Autodesk Inventor part; units mm, degrees
(part 2 of 4)
  line L999 (8.8018, 62.5401) -> (8.8176, 62.5237)
  line L1000 (8.788, 62.5566) -> (8.8018, 62.5401)
  line L1001 (8.7764, 62.5733) -> (8.788, 62.5566)
  line L1002 (8.7669, 62.5901) -> (8.7764, 62.5733)
  line L1003 (8.7595, 62.6071) -> (8.7669, 62.5901)
  line L1004 (8.7542, 62.6241) -> (8.7595, 62.6071)
  line L1005 (8.7511, 62.6412) -> (8.7542, 62.6241)
  line L1006 (8.75, 62.6584) -> (8.7511, 62.6412)
  line L1007 (8.75, 62.8319) -> (8.75, 62.6584)
  line L1008 (8.8777, 62.4763) -> (8.9019, 62.461)
  line L1009 (8.9019, 62.461) -> (8.9282, 62.4462)
  line L1010 (8.9282, 62.4462) -> (8.9566, 62.4317)
  line L1011 (8.9566, 62.4317) -> (8.9871, 62.4176)
  line L1012 (9.0196, 62.4039) -> (9.0542, 62.3907)
  line L1013 (8.9871, 62.4176) -> (9.0196, 62.4039)
  line L1014 (8.7764, 59.9488) -> (8.788, 59.9655)
  line L1015 (8.788, 59.9655) -> (8.8018, 59.9821)
  line L1016 (8.8018, 59.9821) -> (8.8176, 59.9984)
  line L1017 (8.8176, 59.9984) -> (8.8355, 60.0145)
  line L1018 (8.8355, 60.0145) -> (8.8556, 60.0303)
  line L1019 (8.8556, 60.0303) -> (8.8777, 60.0458)
  line L1020 (8.8777, 60.0458) -> (8.9019, 60.0611)
  line L1021 (8.9019, 60.0611) -> (8.9282, 60.0759)
  line L1022 (8.9282, 60.0759) -> (8.9566, 60.0904)
  line L1023 (8.9566, 60.0904) -> (8.9871, 60.1045)
  line L1024 (8.9871, 60.1045) -> (9.0196, 60.1182)
  line L1025 (9.0196, 60.1182) -> (9.0542, 60.1314)
  line L1026 (8.7669, 59.932) -> (8.7764, 59.9488)
  line L1027 (8.7595, 59.915) -> (8.7669, 59.932)
  line L1028 (8.7542, 59.898) -> (8.7595, 59.915)
  line L1029 (8.7511, 59.8809) -> (8.7542, 59.898)
  line L1030 (8.75, 59.8637) -> (8.7511, 59.8809)
  line L1031 (8.75, 59.6903) -> (8.75, 59.8637)
  line L1032 (8.75, 59.6903) -> (8.75, 59.5168)
  line L1033 (8.75, 59.5168) -> (8.7511, 59.4996)
  line L1034 (8.7511, 59.4996) -> (8.7542, 59.4825)
  line L1035 (8.7542, 59.4825) -> (8.7595, 59.4655)
  line L1036 (8.7595, 59.4655) -> (8.7669, 59.4485)
  line L1037 (8.7669, 59.4485) -> (8.7764, 59.4317)
  line L1038 (8.7764, 59.4317) -> (8.788, 59.415)
  line L1039 (8.788, 59.415) -> (8.8018, 59.3985)
  line L1040 (8.8018, 59.3985) -> (8.8176, 59.3821)
  line L1041 (8.8176, 59.3821) -> (8.8355, 59.366)
  line L1042 (8.8556, 59.3502) -> (8.8777, 59.3347)
  line L1043 (8.8355, 59.366) -> (8.8556, 59.3502)
  line L1044 (8.8777, 59.3347) -> (8.9019, 59.3195)
  line L1045 (8.9019, 59.3195) -> (8.9282, 59.3046)
  line L1046 (8.9282, 59.3046) -> (8.9566, 59.2901)
  line L1047 (8.9566, 59.2901) -> (8.9871, 59.276)
  line L1048 (8.9871, 59.276) -> (9.0196, 59.2623)
  line L1049 (9.0196, 59.2623) -> (9.0542, 59.2491)
  line L1050 (9.0542, 59.2491) -> (11, 58.5409)
  line L1051 (11, 58.5409) -> (11, 58.1195)
  line L1052 (9.0542, 56.9898) -> (11, 57.698)
  line L1053 (11, 57.698) -> (11, 58.1195)
  line L1054 (8.8018, 56.8405) -> (8.8176, 56.8568)
  line L1055 (8.8176, 56.8568) -> (8.8355, 56.8729)
  line L1056 (8.8355, 56.8729) -> (8.8556, 56.8887)
  line L1057 (8.8556, 56.8887) -> (8.8777, 56.9043)
  line L1058 (8.8777, 56.9043) -> (8.9019, 56.9195)
  line L1059 (8.9019, 56.9195) -> (8.9282, 56.9344)
  line L1060 (8.9282, 56.9344) -> (8.9566, 56.9489)
  line L1061 (8.9566, 56.9489) -> (8.9871, 56.963)
  line L1062 (8.9871, 56.963) -> (9.0196, 56.9766)
  line L1063 (9.0196, 56.9766) -> (9.0542, 56.9898)
  line L1064 (8.75, 56.5487) -> (8.75, 56.7222)
  line L1065 (8.75, 56.7222) -> (8.7511, 56.7393)
  line L1066 (8.7511, 56.7393) -> (8.7542, 56.7564)
  line L1067 (8.7542, 56.7564) -> (8.7595, 56.7734)
  line L1068 (8.7595, 56.7734) -> (8.7669, 56.7904)
  line L1069 (8.7669, 56.7904) -> (8.7764, 56.8072)
  line L1070 (8.7764, 56.8072) -> (8.788, 56.8239)
  line L1071 (8.788, 56.8239) -> (8.8018, 56.8405)
  line L1072 (8.8777, 56.1931) -> (8.9019, 56.1779)
  line L1073 (8.9019, 56.1779) -> (8.9282, 56.163)
  line L1074 (8.9282, 56.163) -> (8.9566, 56.1485)
  line L1075 (8.9566, 56.1485) -> (8.9871, 56.1344)
  line L1076 (8.7595, 56.3239) -> (8.7669, 56.3069)
  line L1077 (8.7669, 56.3069) -> (8.7764, 56.2901)
  line L1078 (8.7764, 56.2901) -> (8.788, 56.2734)
  line L1079 (8.75, 56.5487) -> (8.75, 56.3752)
  line L1080 (8.75, 56.3752) -> (8.7511, 56.358)
  line L1081 (8.7511, 56.358) -> (8.7542, 56.3409)
  line L1082 (8.7542, 56.3409) -> (8.7595, 56.3239)
  line L1083 (8.788, 56.2734) -> (8.8018, 56.2569)
  line L1084 (8.8018, 56.2569) -> (8.8176, 56.2405)
  line L1085 (8.8355, 56.2245) -> (8.8556, 56.2086)
  line L1086 (8.8556, 56.2086) -> (8.8777, 56.1931)
  line L1087 (8.8176, 56.2405) -> (8.8355, 56.2245)
  line L1088 (8.9871, 56.1344) -> (9.0196, 56.1207)
  line L1089 (9.0196, 56.1207) -> (9.0542, 56.1075)
  line L1090 (9.0542, 56.1075) -> (11, 55.3993)
  line L1091 (11, 55.3993) -> (11, 54.9779)
  line L1092 (9.0542, 53.8482) -> (11, 54.5564)
  line L1093 (11, 54.5564) -> (11, 54.9779)
  line L1094 (8.8777, 53.7627) -> (8.9019, 53.7779)
  line L1095 (8.9019, 53.7779) -> (8.9282, 53.7928)
  line L1096 (8.9282, 53.7928) -> (8.9566, 53.8073)
  line L1097 (8.9566, 53.8073) -> (8.9871, 53.8214)
  line L1098 (8.9871, 53.8214) -> (9.0196, 53.835)
  line L1099 (9.0196, 53.835) -> (9.0542, 53.8482)
  line L1100 (9.0196, 52.9791) -> (9.0542, 52.9659)
  line L1101 (8.9871, 52.9928) -> (9.0196, 52.9791)
  line L1102 (8.9566, 53.0069) -> (8.9871, 52.9928)
  line L1103 (8.9019, 53.0363) -> (8.9282, 53.0214)
  line L1104 (8.8777, 53.0515) -> (8.9019, 53.0363)
  line L1105 (8.8355, 53.0829) -> (8.8556, 53.067)
  line L1106 (8.8176, 53.099) -> (8.8355, 53.0829)
  line L1107 (8.9282, 53.0214) -> (8.9566, 53.0069)
  line L1108 (8.75, 50.2655) -> (8.75, 50.439)
  line L1109 (8.75, 50.439) -> (8.7511, 50.4561)
  line L1110 (8.7511, 50.4561) -> (8.7542, 50.4732)
  line L1111 (8.7542, 50.4732) -> (8.7595, 50.4903)
  line L1112 (8.7595, 50.4903) -> (8.7669, 50.5072)
  line L1113 (8.7669, 50.5072) -> (8.7764, 50.5241)
  line L1114 (8.7764, 50.5241) -> (8.788, 50.5408)
  line L1115 (8.8556, 50.6055) -> (8.8777, 50.6211)
  line L1116 (8.8355, 50.5897) -> (8.8556, 50.6055)
  line L1117 (8.8176, 50.5736) -> (8.8355, 50.5897)
  line L1118 (8.8018, 50.5573) -> (8.8176, 50.5736)
  line L1119 (8.788, 50.5408) -> (8.8018, 50.5573)
  line L1120 (8.8556, 53.067) -> (8.8777, 53.0515)
  line L1121 (9.0542, 60.1314) -> (11, 60.8396)
  line L1122 (11, 60.8396) -> (11, 61.2611)
  line L1123 (11, 61.6825) -> (11, 61.2611)
  line L1124 (9.0542, 62.3907) -> (11, 61.6825)
  line L1125 (8.9282, 88.3503) -> (8.9566, 88.3648)
  line L1126 (8.9566, 88.3648) -> (8.9871, 88.3789)
  line L1127 (8.9871, 88.3789) -> (9.0196, 88.3925)
  line L1128 (8.7669, 88.2063) -> (8.7764, 88.2232)
  line L1129 (8.7764, 88.2232) -> (8.788, 88.2399)
  line L1130 (8.788, 88.2399) -> (8.8018, 88.2564)
  line L1131 (8.8018, 88.2564) -> (8.8176, 88.2727)
  line L1132 (8.8176, 88.2727) -> (8.8355, 88.2888)
  line L1133 (8.8355, 88.2888) -> (8.8556, 88.3046)
  line L1134 (8.8556, 88.3046) -> (8.8777, 88.3202)
  line L1135 (8.8777, 88.3202) -> (8.9019, 88.3354)
  line L1136 (8.9019, 88.3354) -> (8.9282, 88.3503)
  line L1137 (8.75, 87.9646) -> (8.75, 88.1381)
  line L1138 (8.75, 88.1381) -> (8.7511, 88.1552)
  line L1139 (8.7542, 88.1723) -> (8.7595, 88.1894)
  line L1140 (8.7511, 88.1552) -> (8.7542, 88.1723)
  line L1141 (8.75, 87.9646) -> (8.75, 87.7911)
  line L1142 (8.75, 87.7911) -> (8.7511, 87.774)
  line L1143 (8.7511, 87.774) -> (8.7542, 87.7569)
  line L1144 (8.7542, 87.7569) -> (8.7595, 87.7398)
  line L1145 (8.7595, 87.7398) -> (8.7669, 87.7229)
  line L1146 (8.7669, 87.7229) -> (8.7764, 87.706)
  line L1147 (8.7595, 88.1894) -> (8.7669, 88.2063)
  line L1148 (8.9566, 87.5644) -> (8.9871, 87.5503)
  line L1149 (8.9871, 87.5503) -> (9.0196, 87.5366)
  line L1150 (9.0196, 87.5366) -> (9.0542, 87.5234)
  line L1151 (9.0542, 85.2642) -> (11, 85.9724)
  line L1152 (9.0542, 87.5234) -> (11, 86.8152)
  line L1153 (11, 85.9724) -> (11, 86.3938)
  line L1154 (11, 86.8152) -> (11, 86.3938)
  line L1155 (8.9282, 87.5789) -> (8.9566, 87.5644)
  line L1156 (8.9019, 87.5938) -> (8.9282, 87.5789)
  line L1157 (8.8777, 87.609) -> (8.9019, 87.5938)
  line L1158 (8.8556, 87.6246) -> (8.8777, 87.609)
  line L1159 (8.8355, 87.6404) -> (8.8556, 87.6246)
  line L1160 (8.8176, 87.6565) -> (8.8355, 87.6404)
  line L1161 (8.8018, 87.6728) -> (8.8176, 87.6565)
  line L1162 (8.7764, 87.706) -> (8.788, 87.6893)
  line L1163 (8.788, 87.6893) -> (8.8018, 87.6728)
  line L1164 (8.8018, 85.1148) -> (8.8176, 85.1311)
  line L1165 (8.788, 85.0983) -> (8.8018, 85.1148)
  line L1166 (8.7764, 85.0816) -> (8.788, 85.0983)
  line L1167 (8.7669, 85.0647) -> (8.7764, 85.0816)
  line L1168 (8.7595, 85.0478) -> (8.7669, 85.0647)
  line L1169 (8.7511, 85.0136) -> (8.7542, 85.0307)
  line L1170 (8.75, 84.9965) -> (8.7511, 85.0136)
  line L1171 (8.75, 84.823) -> (8.75, 84.9965)
  line L1172 (8.7542, 85.0307) -> (8.7595, 85.0478)
  line L1173 (8.75, 84.823) -> (8.75, 84.6495)
  line L1174 (8.75, 84.6495) -> (8.7511, 84.6324)
  line L1175 (8.7511, 84.6324) -> (8.7542, 84.6153)
  line L1176 (8.7542, 84.6153) -> (8.7595, 84.5982)
  line L1177 (8.7595, 84.5982) -> (8.7669, 84.5813)
  line L1178 (8.7669, 84.5813) -> (8.7764, 84.5644)
  line L1179 (8.7764, 84.5644) -> (8.788, 84.5477)
  line L1180 (8.788, 84.5477) -> (8.8018, 84.5312)
  line L1181 (8.8018, 84.5312) -> (8.8176, 84.5149)
  line L1182 (8.8355, 84.4988) -> (8.8556, 84.483)
  line L1183 (8.8556, 84.483) -> (8.8777, 84.4674)
  line L1184 (8.8777, 84.4674) -> (8.9019, 84.4522)
  line L1185 (8.9019, 84.4522) -> (8.9282, 84.4373)
  line L1186 (8.9282, 84.4373) -> (8.9566, 84.4228)
  line L1187 (8.8176, 84.5149) -> (8.8355, 84.4988)
  line L1188 (8.9871, 84.4087) -> (9.0196, 84.395)
  line L1189 (9.0196, 84.395) -> (9.0542, 84.3818)
  line L1190 (9.0542, 84.3818) -> (11, 83.6736)
  line L1191 (11, 83.6736) -> (11, 83.2522)
  line L1192 (11, 82.8308) -> (11, 83.2522)
  line L1193 (9.0542, 82.1226) -> (11, 82.8308)
  line L1194 (8.9566, 84.4228) -> (8.9871, 84.4087)
  line L1195 (8.8777, 82.037) -> (8.9019, 82.0522)
  line L1196 (8.9019, 82.0522) -> (8.9282, 82.0671)
  line L1197 (8.9282, 82.0671) -> (8.9566, 82.0816)
  line L1198 (8.9871, 82.0957) -> (9.0196, 82.1094)
  line L1199 (9.0196, 82.1094) -> (9.0542, 82.1226)
  line L1200 (8.9566, 82.0816) -> (8.9871, 82.0957)
  line L1201 (8.75, 81.6814) -> (8.75, 81.8549)
  line L1202 (8.75, 81.8549) -> (8.7511, 81.872)
  line L1203 (8.7511, 81.872) -> (8.7542, 81.8891)
  line L1204 (8.7542, 81.8891) -> (8.7595, 81.9062)
  line L1205 (8.7595, 81.9062) -> (8.7669, 81.9231)
  line L1206 (8.7669, 81.9231) -> (8.7764, 81.94)
  line L1207 (8.7764, 81.94) -> (8.788, 81.9567)
  line L1208 (8.788, 81.9567) -> (8.8018, 81.9732)
  line L1209 (8.8018, 81.9732) -> (8.8176, 81.9895)
  line L1210 (8.8176, 81.9895) -> (8.8355, 82.0056)
  line L1211 (8.8355, 82.0056) -> (8.8556, 82.0215)
  line L1212 (8.8556, 82.0215) -> (8.8777, 82.037)
  line L1213 (8.8777, 81.3258) -> (8.9019, 81.3106)
  line L1214 (8.9019, 81.3106) -> (8.9282, 81.2957)
  line L1215 (8.75, 81.6814) -> (8.75, 81.5079)
  line L1216 (8.75, 81.5079) -> (8.7511, 81.4908)
  line L1217 (8.7511, 81.4908) -> (8.7542, 81.4737)
  line L1218 (8.7542, 81.4737) -> (8.7595, 81.4566)
  line L1219 (8.8556, 81.3414) -> (8.8777, 81.3258)
  line L1220 (8.8355, 81.3572) -> (8.8556, 81.3414)
  line L1221 (8.8176, 81.3733) -> (8.8355, 81.3572)
  line L1222 (8.7669, 81.4397) -> (8.7764, 81.4228)
  line L1223 (8.7764, 81.4228) -> (8.788, 81.4061)
  line L1224 (8.788, 81.4061) -> (8.8018, 81.3896)
  line L1225 (8.8018, 81.3896) -> (8.8176, 81.3733)
  line L1226 (8.7595, 81.4566) -> (8.7669, 81.4397)
  line L1227 (9.0196, 81.2535) -> (9.0542, 81.2402)
  line L1228 (8.9871, 81.2671) -> (9.0196, 81.2535)
  line L1229 (8.9282, 81.2957) -> (8.9566, 81.2812)
  line L1230 (8.9566, 81.2812) -> (8.9871, 81.2671)
  line L1231 (8.9871, 78.9541) -> (9.0196, 78.9678)
  line L1232 (9.0196, 78.9678) -> (9.0542, 78.981)
  line L1233 (9.0542, 78.981) -> (11, 79.6892)
  line L1234 (11, 79.6892) -> (11, 80.1106)
  line L1235 (11, 80.532) -> (11, 80.1106)
  line L1236 (9.0542, 81.2402) -> (11, 80.532)
  line L1237 (8.9566, 78.94) -> (8.9871, 78.9541)
  line L1238 (8.7764, 78.7984) -> (8.788, 78.8151)
  line L1239 (8.8018, 78.8316) -> (8.8176, 78.8479)
  line L1240 (8.8176, 78.8479) -> (8.8355, 78.864)
  line L1241 (8.8355, 78.864) -> (8.8556, 78.8799)
  line L1242 (8.8556, 78.8799) -> (8.8777, 78.8954)
  line L1243 (8.8777, 78.8954) -> (8.9019, 78.9106)
  line L1244 (8.9019, 78.9106) -> (8.9282, 78.9255)
  line L1245 (8.9282, 78.9255) -> (8.9566, 78.94)
  line L1246 (8.788, 78.8151) -> (8.8018, 78.8316)
  line L1247 (8.75, 78.5398) -> (8.75, 78.7133)
  line L1248 (8.75, 78.7133) -> (8.7511, 78.7304)
  line L1249 (8.7511, 78.7304) -> (8.7542, 78.7475)
  line L1250 (8.7595, 78.7646) -> (8.7669, 78.7815)
  line L1251 (8.7669, 78.7815) -> (8.7764, 78.7984)
  line L1252 (8.7542, 78.7475) -> (8.7595, 78.7646)
  line L1253 (8.788, 78.2645) -> (8.8018, 78.248)
  line L1254 (8.7764, 78.2812) -> (8.788, 78.2645)
  line L1255 (8.7669, 78.2981) -> (8.7764, 78.2812)
  line L1256 (8.7595, 78.315) -> (8.7669, 78.2981)
  line L1257 (8.7542, 78.3321) -> (8.7595, 78.315)
  line L1258 (8.7511, 78.3492) -> (8.7542, 78.3321)
  line L1259 (8.75, 78.3663) -> (8.7511, 78.3492)
  line L1260 (8.75, 78.5398) -> (8.75, 78.3663)
  line L1261 (8.9871, 75.8125) -> (9.0196, 75.8262)
  line L1262 (9.0196, 75.8262) -> (9.0542, 75.8394)
  line L1263 (9.0542, 75.8394) -> (11, 76.5476)
  line L1264 (11, 76.5476) -> (11, 76.969)
  line L1265 (11, 77.3904) -> (11, 76.969)
  line L1266 (9.0542, 78.0987) -> (11, 77.3904)
  line L1267 (9.0196, 78.1119) -> (9.0542, 78.0987)
  line L1268 (8.8018, 78.248) -> (8.8176, 78.2317)
  line L1269 (8.8176, 78.2317) -> (8.8355, 78.2156)
  line L1270 (8.8355, 78.2156) -> (8.8556, 78.1998)
  line L1271 (8.8556, 78.1998) -> (8.8777, 78.1842)
  line L1272 (8.8777, 78.1842) -> (8.9019, 78.169)
  line L1273 (8.9019, 78.169) -> (8.9282, 78.1541)
  line L1274 (8.9282, 78.1541) -> (8.9566, 78.1396)
  line L1275 (8.9566, 78.1396) -> (8.9871, 78.1255)
  line L1276 (8.9871, 78.1255) -> (9.0196, 78.1119)
  line L1277 (8.8176, 85.1311) -> (8.8355, 85.1472)
  line L1278 (8.8355, 85.1472) -> (8.8556, 85.163)
  line L1279 (8.8556, 85.163) -> (8.8777, 85.1786)
  line L1280 (8.8777, 85.1786) -> (8.9019, 85.1938)
  line L1281 (8.9019, 85.1938) -> (8.9282, 85.2087)
  line L1282 (8.9282, 85.2087) -> (8.9566, 85.2232)
  line L1283 (8.9566, 85.2232) -> (8.9871, 85.2373)
  line L1284 (8.9871, 85.2373) -> (9.0196, 85.251)
  line L1285 (9.0196, 85.251) -> (9.0542, 85.2642)
  line L1286 (-1.25, 99.281) -> (-1.25, 109.281)
  line L1287 (-1.25, 109.281) -> (8.75, 109.281)
  line L1288 (8.75, 109.281) -> (8.75, 100.531)
  line L1289 (9.6684, 106.1616) -> (10.0504, 106.1616)
  line L1290 (10.0504, 106.1616) -> (10.0504, 106.0668)
  line L1291 (10.0504, 106.0668) -> (9.6684, 106.0668)
  line L1292 (9.6684, 106.0668) -> (9.6684, 106.1616)
  line L1293 (-2.25, 0) -> (-1.25, 0)
  line L1294 (8.75, 0) -> (12, 0)
  line L1295 (-1.25, 99.281) -> (-1.25, 10.75)
  line L1296 (8.7511, -56.358) -> (8.7542, -56.3409)
  line L1297 (8.7542, -56.3409) -> (8.7595, -56.3239)
  line L1298 (8.7595, -56.3239) -> (8.7669, -56.3069)
  line L1299 (8.7669, -56.3069) -> (8.7764, -56.2901)
  line L1300 (8.7764, -56.2901) -> (8.788, -56.2734)
  line L1301 (8.788, -56.2734) -> (8.8018, -56.2569)
  line L1302 (8.8018, -56.2569) -> (8.8176, -56.2405)
  line L1303 (8.8176, -56.2405) -> (8.8355, -56.2245)
  line L1304 (8.8355, -56.2245) -> (8.8556, -56.2086)
  line L1305 (8.8556, -56.2086) -> (8.8777, -56.1931)
  line L1306 (8.8777, -56.1931) -> (8.9019, -56.1779)
  line L1307 (8.9019, -56.1779) -> (8.9282, -56.163)
  line L1308 (8.9282, -56.163) -> (8.9566, -56.1485)
  line L1309 (8.9566, -56.1485) -> (8.9871, -56.1344)
  line L1310 (8.788, -56.8239) -> (8.8018, -56.8405)
  line L1311 (8.7764, -56.8072) -> (8.788, -56.8239)
  line L1312 (8.7669, -56.7904) -> (8.7764, -56.8072)
  line L1313 (8.7595, -56.7734) -> (8.7669, -56.7904)
  line L1314 (8.7542, -56.7564) -> (8.7595, -56.7734)
  line L1315 (8.75, -56.7222) -> (8.7511, -56.7393)
  line L1316 (8.75, -56.5487) -> (8.75, -56.7222)
  line L1317 (8.75, -56.5487) -> (8.75, -56.3752)
  line L1318 (8.75, -56.3752) -> (8.7511, -56.358)
  line L1319 (8.7511, -56.7393) -> (8.7542, -56.7564)
  line L1320 (9.0196, -56.9766) -> (9.0542, -56.9898)
  line L1321 (8.9871, -56.963) -> (9.0196, -56.9766)
  line L1322 (8.9566, -56.9489) -> (8.9871, -56.963)
  line L1323 (8.9282, -56.9344) -> (8.9566, -56.9489)
  line L1324 (8.9019, -56.9195) -> (8.9282, -56.9344)
  line L1325 (8.8777, -56.9043) -> (8.9019, -56.9195)
  line L1326 (8.8355, -56.8729) -> (8.8556, -56.8887)
  line L1327 (8.8176, -56.8568) -> (8.8355, -56.8729)
  line L1328 (8.8018, -56.8405) -> (8.8176, -56.8568)
  line L1329 (8.8556, -56.8887) -> (8.8777, -56.9043)
  line L1330 (8.8018, -59.3985) -> (8.8176, -59.3821)
  line L1331 (8.8176, -59.3821) -> (8.8355, -59.366)
  line L1332 (8.8556, -59.3502) -> (8.8777, -59.3347)
  line L1333 (8.8355, -59.366) -> (8.8556, -59.3502)
  line L1334 (8.8777, -59.3347) -> (8.9019, -59.3195)
  line L1335 (8.9019, -59.3195) -> (8.9282, -59.3046)
  line L1336 (8.9282, -59.3046) -> (8.9566, -59.2901)
  line L1337 (9.0542, -56.9898) -> (11, -57.698)
  line L1338 (11, -57.698) -> (11, -58.1195)
  line L1339 (8.9566, -59.2901) -> (8.9871, -59.276)
  line L1340 (8.9871, -59.276) -> (9.0196, -59.2623)
  line L1341 (11, -58.5409) -> (11, -58.1195)
  line L1342 (9.0542, -59.2491) -> (11, -58.5409)
  line L1343 (9.0196, -59.2623) -> (9.0542, -59.2491)
  line L1344 (8.788, -59.415) -> (8.8018, -59.3985)
  line L1345 (8.7764, -59.4317) -> (8.788, -59.415)
  line L1346 (8.7669, -59.4485) -> (8.7764, -59.4317)
  line L1347 (8.7595, -59.4655) -> (8.7669, -59.4485)
  line L1348 (8.7542, -59.4825) -> (8.7595, -59.4655)
  line L1349 (8.7511, -59.4996) -> (8.7542, -59.4825)
  line L1350 (8.75, -59.5168) -> (8.7511, -59.4996)
  line L1351 (8.75, -59.6903) -> (8.75, -59.5168)
  line L1352 (8.75, -59.6903) -> (8.75, -59.8637)
  line L1353 (8.7511, -59.8809) -> (8.7542, -59.898)
  line L1354 (8.7542, -59.898) -> (8.7595, -59.915)
  line L1355 (8.7595, -59.915) -> (8.7669, -59.932)
  line L1356 (8.7669, -59.932) -> (8.7764, -59.9488)
  line L1357 (8.75, -59.8637) -> (8.7511, -59.8809)
  line L1358 (8.9871, -60.1045) -> (9.0196, -60.1182)
  line L1359 (8.9566, -60.0904) -> (8.9871, -60.1045)
  line L1360 (8.9282, -60.0759) -> (8.9566, -60.0904)
  line L1361 (8.9019, -60.0611) -> (8.9282, -60.0759)
  line L1362 (8.8777, -60.0458) -> (8.9019, -60.0611)
  line L1363 (8.8556, -60.0303) -> (8.8777, -60.0458)
  line L1364 (8.8355, -60.0145) -> (8.8556, -60.0303)
  line L1365 (8.8176, -59.9984) -> (8.8355, -60.0145)
  line L1366 (8.8018, -59.9821) -> (8.8176, -59.9984)
  line L1367 (8.788, -59.9655) -> (8.8018, -59.9821)
  line L1368 (8.7764, -59.9488) -> (8.788, -59.9655)
  line L1369 (8.7764, -63.0904) -> (8.788, -63.1071)
  line L1370 (8.8018, -63.1237) -> (8.8176, -63.14)
  line L1371 (8.8176, -63.14) -> (8.8355, -63.1561)
  line L1372 (8.788, -63.1071) -> (8.8018, -63.1237)
  line L1373 (8.8556, -62.4918) -> (8.8777, -62.4763)
  line L1374 (8.8355, -62.5076) -> (8.8556, -62.4918)
  line L1375 (8.8176, -62.5237) -> (8.8355, -62.5076)
  line L1376 (8.8018, -62.5401) -> (8.8176, -62.5237)
  line L1377 (8.788, -62.5566) -> (8.8018, -62.5401)
  line L1378 (8.7764, -62.5733) -> (8.788, -62.5566)
  line L1379 (8.7669, -62.5901) -> (8.7764, -62.5733)
  line L1380 (8.7542, -62.6241) -> (8.7595, -62.6071)
  line L1381 (8.7511, -62.6412) -> (8.7542, -62.6241)
  line L1382 (8.75, -62.6584) -> (8.7511, -62.6412)
  line L1383 (8.75, -62.8319) -> (8.75, -62.6584)
  line L1384 (8.7595, -62.6071) -> (8.7669, -62.5901)
  line L1385 (8.75, -65.9734) -> (8.75, -66.1469)
  line L1386 (8.75, -66.1469) -> (8.7511, -66.1641)
  line L1387 (8.7595, -68.8903) -> (8.7669, -68.8733)
  line L1388 (8.7542, -68.9073) -> (8.7595, -68.8903)
  line L1389 (8.7511, -68.9244) -> (8.7542, -68.9073)
  line L1390 (8.75, -68.9416) -> (8.7511, -68.9244)
  line L1391 (8.75, -69.115) -> (8.75, -68.9416)
  line L1392 (8.75, -75.3982) -> (7.9383, -75.3982)
  line L1393 (8.7669, -68.8733) -> (8.7764, -68.8565)
  line L1394 (8.7595, -90.8814) -> (8.7669, -90.8645)
  line L1395 (8.7511, -90.9156) -> (8.7542, -90.8985)
  line L1396 (8.7542, -90.8985) -> (8.7595, -90.8814)
  line L1397 (8.8777, -62.4763) -> (8.9019, -62.461)
  line L1398 (8.9019, -62.461) -> (8.9282, -62.4462)
  line L1399 (8.9282, -62.4462) -> (8.9566, -62.4317)
  line L1400 (8.9566, -62.4317) -> (8.9871, -62.4176)
  line L1401 (9.0196, -62.4039) -> (9.0542, -62.3907)
  line L1402 (9.0542, -60.1314) -> (11, -60.8396)
  line L1403 (8.9871, -62.4176) -> (9.0196, -62.4039)
  line L1404 (11, -60.8396) -> (11, -61.2611)
  line L1405 (11, -61.6825) -> (11, -61.2611)
  line L1406 (9.0542, -62.3907) -> (11, -61.6825)
  line L1407 (9.0196, -60.1182) -> (9.0542, -60.1314)
  line L1408 (8.8176, -12.2583) -> (8.8355, -12.2422)
  line L1409 (8.8018, -12.2746) -> (8.8176, -12.2583)
  line L1410 (8.788, -12.2911) -> (8.8018, -12.2746)
  line L1411 (8.7764, -12.3078) -> (8.788, -12.2911)
  line L1412 (8.7669, -12.3246) -> (8.7764, -12.3078)
  line L1413 (8.7595, -12.3416) -> (8.7669, -12.3246)
  line L1414 (8.7542, -12.3586) -> (8.7595, -12.3416)
  line L1415 (8.7511, -12.3758) -> (8.7542, -12.3586)
  line L1416 (8.75, -12.3929) -> (8.7511, -12.3758)
  line L1417 (8.75, -12.5664) -> (8.75, -12.3929)
  line L1418 (8.75, -12.5664) -> (7.1265, -12.5664)
  line L1419 (8.9282, -12.1807) -> (8.9566, -12.1662)
  line L1420 (8.9566, -12.1662) -> (8.9871, -12.1521)
  line L1421 (8.9871, -12.1521) -> (9.0196, -12.1384)
  line L1422 (9.0196, -12.1384) -> (9.0542, -12.1252)
  line L1423 (8.8355, -12.2422) -> (8.8556, -12.2263)
  line L1424 (8.8556, -12.2263) -> (8.8777, -12.2108)
  line L1425 (8.8777, -12.2108) -> (8.9019, -12.1956)
  line L1426 (8.9019, -12.1956) -> (8.9282, -12.1807)
  line L1427 (9.0542, -12.1252) -> (11, -11.417)
  line L1428 (11, -11.417) -> (11, -10.9956)
  line L1429 (8.75, -25.1327) -> (8.75, -24.9593)
  line L1430 (9.0542, -53.8482) -> (11, -54.5564)
  line L1431 (11, -54.5564) -> (11, -54.9779)
  line L1432 (9.0196, -56.1207) -> (9.0542, -56.1075)
  line L1433 (11, -55.3993) -> (11, -54.9779)
  line L1434 (9.0542, -56.1075) -> (11, -55.3993)
  line L1435 (8.9871, -56.1344) -> (9.0196, -56.1207)
  line L1436 (8.7542, -40.633) -> (8.7595, -40.6159)
  line L1437 (8.7511, -40.6501) -> (8.7542, -40.633)
  line L1438 (8.75, -40.6672) -> (8.7511, -40.6501)
  line L1439 (8.75, -40.8407) -> (8.75, -40.6672)
  line L1440 (8.75, -40.8407) -> (8.75, -41.0142)
  line L1441 (8.75, -41.0142) -> (8.7511, -41.0313)
  line L1442 (8.7511, -41.0313) -> (8.7542, -41.0484)
  line L1443 (8.7542, -41.0484) -> (8.7595, -41.0655)
  line L1444 (8.7542, -50.0578) -> (8.7595, -50.0407)
  line L1445 (8.75, -50.092) -> (8.7511, -50.0749)
  line L1446 (8.7764, -53.6656) -> (8.788, -53.6823)
  line L1447 (8.9871, -53.8214) -> (9.0196, -53.835)
  line L1448 (8.9566, -53.8073) -> (8.9871, -53.8214)
  line L1449 (8.9282, -53.7928) -> (8.9566, -53.8073)
  line L1450 (8.9019, -53.7779) -> (8.9282, -53.7928)
  line L1451 (8.8777, -53.7627) -> (8.9019, -53.7779)
  line L1452 (8.8556, -53.7471) -> (8.8777, -53.7627)
  line L1453 (8.8355, -53.7313) -> (8.8556, -53.7471)
  line L1454 (8.8176, -53.7152) -> (8.8355, -53.7313)
  line L1455 (8.8018, -53.6989) -> (8.8176, -53.7152)
  line L1456 (8.788, -53.6823) -> (8.8018, -53.6989)
  line L1457 (9.0196, -53.835) -> (9.0542, -53.8482)
  line L1458 (8.7669, -53.6488) -> (8.7764, -53.6656)
  line L1459 (8.7595, -53.6318) -> (8.7669, -53.6488)
  line L1460 (8.7542, -53.6148) -> (8.7595, -53.6318)
  line L1461 (8.7511, -53.5977) -> (8.7542, -53.6148)
  line L1462 (8.75, -53.5806) -> (8.7511, -53.5977)
  line L1463 (8.75, -53.4071) -> (8.75, -53.5806)
  line L1464 (8.75, -53.4071) -> (8.75, -53.2336)
  line L1465 (8.75, -53.2336) -> (8.7511, -53.2165)
  line L1466 (8.7511, -53.2165) -> (8.7542, -53.1994)
  line L1467 (8.7542, -53.1994) -> (8.7595, -53.1823)
  line L1468 (8.7595, -53.1823) -> (8.7669, -53.1653)
  line L1469 (8.7669, -53.1653) -> (8.7764, -53.1485)
  line L1470 (8.788, -53.1318) -> (8.8018, -53.1153)
  line L1471 (8.8018, -53.1153) -> (8.8176, -53.099)
  line L1472 (8.7764, -53.1485) -> (8.788, -53.1318)
  line L1473 (8.9871, -52.9928) -> (9.0196, -52.9791)
  line L1474 (9.0196, -52.9791) -> (9.0542, -52.9659)
  line L1475 (8.9566, -53.0069) -> (8.9871, -52.9928)
  line L1476 (8.9282, -53.0214) -> (8.9566, -53.0069)
  line L1477 (8.9019, -53.0363) -> (8.9282, -53.0214)
  line L1478 (8.8777, -53.0515) -> (8.9019, -53.0363)
  line L1479 (8.8556, -53.067) -> (8.8777, -53.0515)
  line L1480 (8.8176, -53.099) -> (8.8355, -53.0829)
  line L1481 (8.8355, -53.0829) -> (8.8556, -53.067)
  line L1482 (8.9019, -50.6363) -> (8.9282, -50.6512)
  line L1483 (9.0542, -52.9659) -> (11, -52.2577)
  line L1484 (11, -52.2577) -> (11, -51.8363)
  line L1485 (11, -51.4149) -> (11, -51.8363)
  line L1486 (9.0542, -50.7066) -> (11, -51.4149)
  line L1487 (8.7595, -50.4903) -> (8.7669, -50.5072)
  line L1488 (8.7764, -50.5241) -> (8.788, -50.5408)
  line L1489 (8.788, -50.5408) -> (8.8018, -50.5573)
  line L1490 (8.8018, -50.5573) -> (8.8176, -50.5736)
  line L1491 (8.8176, -50.5736) -> (8.8355, -50.5897)
  line L1492 (8.8355, -50.5897) -> (8.8556, -50.6055)
  line L1493 (8.8556, -50.6055) -> (8.8777, -50.6211)
  line L1494 (8.8777, -50.6211) -> (8.9019, -50.6363)
  line L1495 (8.9282, -50.6512) -> (8.9566, -50.6657)
  line L1496 (8.9566, -50.6657) -> (8.9871, -50.6798)
  line L1497 (9.0196, -50.6934) -> (9.0542, -50.7066)
  line L1498 (8.9871, -50.6798) -> (9.0196, -50.6934)
  line L1499 (8.75, -50.2655) -> (8.75, -50.439)
  line L1500 (8.75, -50.439) -> (8.7511, -50.4561)
  line L1501 (8.7511, -50.4561) -> (8.7542, -50.4732)
  line L1502 (8.7542, -50.4732) -> (8.7595, -50.4903)
  line L1503 (8.7669, -50.5072) -> (8.7764, -50.5241)
  line L1504 (8.75, -50.2655) -> (8.75, -50.092)
  line L1505 (8.7511, -50.0749) -> (8.7542, -50.0578)
  line L1506 (8.7595, -50.0407) -> (8.7669, -50.0238)
  line L1507 (8.7669, -50.0238) -> (8.7764, -50.0069)
  line L1508 (8.7764, -50.0069) -> (8.788, -49.9902)
  line L1509 (8.788, -49.9902) -> (8.8018, -49.9737)
  line L1510 (8.8018, -49.9737) -> (8.8176, -49.9574)
  line L1511 (8.8176, -49.9574) -> (8.8355, -49.9413)
  line L1512 (8.8355, -49.9413) -> (8.8556, -49.9254)
  line L1513 (8.8556, -49.9254) -> (8.8777, -49.9099)
  line L1514 (8.8777, -49.9099) -> (8.9019, -49.8947)
  line L1515 (8.9019, -49.8947) -> (8.9282, -49.8798)
  line L1516 (8.9282, -49.8798) -> (8.9566, -49.8653)
  line L1517 (8.9566, -49.8653) -> (8.9871, -49.8512)
  line L1518 (8.9871, -49.8512) -> (9.0196, -49.8375)
  line L1519 (8.75, -24.9593) -> (8.7511, -24.9421)
  line L1520 (8.7511, -24.9421) -> (8.7542, -24.925)
  line L1521 (8.7542, -24.925) -> (8.7595, -24.908)
  line L1522 (8.7595, -24.908) -> (8.7669, -24.891)
  line L1523 (8.7669, -24.891) -> (8.7764, -24.8742)
  line L1524 (8.7764, -24.8742) -> (8.788, -24.8575)
  line L1525 (8.788, -24.8575) -> (8.8018, -24.8409)
  line L1526 (8.8018, -24.8409) -> (8.8176, -24.8246)
  line L1527 (8.9871, -24.7185) -> (9.0196, -24.7048)
  line L1528 (9.0196, -24.7048) -> (9.0542, -24.6916)
  line L1529 (8.9566, -24.7326) -> (8.9871, -24.7185)
  line L1530 (8.9282, -24.7471) -> (8.9566, -24.7326)
  line L1531 (8.9019, -24.7619) -> (8.9282, -24.7471)
  line L1532 (8.8777, -24.7772) -> (8.9019, -24.7619)
  line L1533 (8.8355, -24.8085) -> (8.8556, -24.7927)
  line L1534 (8.8176, -24.8246) -> (8.8355, -24.8085)
  line L1535 (8.8556, -24.7927) -> (8.8777, -24.7772)
  line L1536 (9.0542, -24.6916) -> (11, -23.9834)
  line L1537 (11, -23.9834) -> (11, -23.5619)
  line L1538 (11, -23.1405) -> (11, -23.5619)
  line L1539 (9.0542, -22.4323) -> (11, -23.1405)
  line L1540 (9.0196, -22.4191) -> (9.0542, -22.4323)
  line L1541 (8.9871, -22.4054) -> (9.0196, -22.4191)
  line L1542 (8.9566, -22.3913) -> (8.9871, -22.4054)
  line L1543 (8.9019, -22.362) -> (8.9282, -22.3768)
  line L1544 (8.8777, -22.3467) -> (8.9019, -22.362)
  line L1545 (8.8556, -22.3312) -> (8.8777, -22.3467)
  line L1546 (8.8355, -22.3154) -> (8.8556, -22.3312)
  line L1547 (8.8176, -22.2993) -> (8.8355, -22.3154)
  line L1548 (8.9282, -22.3768) -> (8.9566, -22.3913)
  line L1549 (8.8018, -22.2829) -> (8.8176, -22.2993)
  line L1550 (8.788, -22.2664) -> (8.8018, -22.2829)
  line L1551 (8.7764, -22.2497) -> (8.788, -22.2664)
  line L1552 (8.7669, -22.2329) -> (8.7764, -22.2497)
  line L1553 (8.7595, -22.2159) -> (8.7669, -22.2329)
  line L1554 (8.7542, -22.1989) -> (8.7595, -22.2159)
  line L1555 (8.7511, -22.1818) -> (8.7542, -22.1989)
  line L1556 (8.75, -22.1646) -> (8.7511, -22.1818)
  line L1557 (8.7764, -21.7326) -> (8.788, -21.7159)
  line L1558 (8.788, -21.7159) -> (8.8018, -21.6994)
  line L1559 (8.8018, -21.6994) -> (8.8176, -21.683)
  line L1560 (8.8355, -21.6669) -> (8.8556, -21.6511)
  line L1561 (8.8556, -21.6511) -> (8.8777, -21.6356)
  line L1562 (8.8777, -21.6356) -> (8.9019, -21.6203)
  line L1563 (8.9019, -21.6203) -> (8.9282, -21.6055)
  line L1564 (8.9282, -21.6055) -> (8.9566, -21.591)
  line L1565 (8.8176, -21.683) -> (8.8355, -21.6669)
  line L1566 (9.0196, -21.5632) -> (9.0542, -21.55)
  line L1567 (8.9871, -21.5769) -> (9.0196, -21.5632)
  line L1568 (8.7542, -21.7834) -> (8.7595, -21.7664)
  line L1569 (8.9566, -21.591) -> (8.9871, -21.5769)
  line L1570 (9.0542, -21.55) -> (11, -20.8418)
  line L1571 (11, -20.8418) -> (11, -20.4204)
  line L1572 (11, -19.9989) -> (11, -20.4204)
  line L1573 (9.0542, -19.2907) -> (11, -19.9989)
  line L1574 (9.0196, -19.2775) -> (9.0542, -19.2907)
  line L1575 (8.9871, -19.2638) -> (9.0196, -19.2775)
  line L1576 (8.9566, -19.2497) -> (8.9871, -19.2638)
  line L1577 (8.9282, -19.2352) -> (8.9566, -19.2497)
  line L1578 (8.9019, -19.2204) -> (8.9282, -19.2352)
  line L1579 (8.8777, -19.2051) -> (8.9019, -19.2204)
  line L1580 (8.8556, -19.1896) -> (8.8777, -19.2051)
  line L1581 (8.8355, -19.1738) -> (8.8556, -19.1896)
  line L1582 (8.8176, -19.1577) -> (8.8355, -19.1738)
  line L1583 (8.8018, -19.1414) -> (8.8176, -19.1577)
  line L1584 (8.788, -19.1248) -> (8.8018, -19.1414)
  line L1585 (8.7764, -19.1081) -> (8.788, -19.1248)
  line L1586 (8.7669, -19.0913) -> (8.7764, -19.1081)
  line L1587 (8.7595, -19.0743) -> (8.7669, -19.0913)
  line L1588 (8.7542, -19.0573) -> (8.7595, -19.0743)
  line L1589 (8.7511, -19.0402) -> (8.7542, -19.0573)
  line L1590 (8.75, -21.9911) -> (8.75, -22.1646)
  line L1591 (8.75, -19.023) -> (8.7511, -19.0402)
  line L1592 (8.75, -18.8496) -> (8.75, -19.023)
  line L1593 (9.0196, -49.8375) -> (9.0542, -49.8243)
  line L1594 (9.0542, -49.8243) -> (11, -49.1161)
  line L1595 (9.0542, -47.5651) -> (11, -48.2733)
  line L1596 (11, -48.2733) -> (11, -48.6947)
  line L1597 (11, -49.1161) -> (11, -48.6947)
  line L1598 (8.788, -47.3992) -> (8.8018, -47.4157)
  line L1599 (8.7764, -47.3825) -> (8.788, -47.3992)
  line L1600 (8.7669, -47.3656) -> (8.7764, -47.3825)
  line L1601 (8.75, -47.1239) -> (8.75, -47.2974)
  line L1602 (8.75, -47.2974) -> (8.7511, -47.3145)
  line L1603 (8.7511, -47.3145) -> (8.7542, -47.3316)
  line L1604 (8.7542, -47.3316) -> (8.7595, -47.3487)
  line L1605 (8.7595, -47.3487) -> (8.7669, -47.3656)
  line L1606 (8.75, -47.1239) -> (8.75, -46.9504)
  line L1607 (8.75, -46.9504) -> (8.7511, -46.9333)
  line L1608 (8.7511, -46.9333) -> (8.7542, -46.9162)
  line L1609 (8.7542, -46.9162) -> (8.7595, -46.8991)
  line L1610 (8.7595, -46.8991) -> (8.7669, -46.8822)
  line L1611 (8.7669, -46.8822) -> (8.7764, -46.8653)
  line L1612 (8.7764, -46.8653) -> (8.788, -46.8486)
  line L1613 (8.788, -46.8486) -> (8.8018, -46.8321)
  line L1614 (8.8018, -46.8321) -> (8.8176, -46.8158)
  line L1615 (8.8176, -46.8158) -> (8.8355, -46.7997)
  line L1616 (8.8355, -46.7997) -> (8.8556, -46.7838)
  line L1617 (8.8556, -46.7838) -> (8.8777, -46.7683)
  line L1618 (8.8777, -44.3379) -> (8.9019, -44.3531)
  line L1619 (8.9019, -44.3531) -> (8.9282, -44.368)
  line L1620 (8.788, -44.2576) -> (8.8018, -44.2741)
  line L1621 (8.8018, -44.2741) -> (8.8176, -44.2904)
  line L1622 (8.8176, -44.2904) -> (8.8355, -44.3065)
  line L1623 (8.8355, -44.3065) -> (8.8556, -44.3223)
  line L1624 (8.8556, -44.3223) -> (8.8777, -44.3379)
  line L1625 (8.9282, -44.368) -> (8.9566, -44.3825)
  line L1626 (8.9871, -44.3966) -> (9.0196, -44.4103)
  line L1627 (9.0196, -44.4103) -> (9.0542, -44.4235)
  line L1628 (8.9566, -44.3825) -> (8.9871, -44.3966)
  line L1629 (8.7764, -44.2409) -> (8.788, -44.2576)
  line L1630 (8.7669, -44.224) -> (8.7764, -44.2409)
  line L1631 (8.7595, -44.2071) -> (8.7669, -44.224)
  line L1632 (8.75, -44.1558) -> (8.7511, -44.1729)
  line L1633 (8.75, -43.9823) -> (8.75, -44.1558)
  line L1634 (8.75, -43.9823) -> (8.75, -43.8088)
  line L1635 (8.75, -43.8088) -> (8.7511, -43.7917)
  line L1636 (8.9019, -46.7531) -> (8.9282, -46.7382)
  line L1637 (8.9282, -46.7382) -> (8.9566, -46.7237)
  line L1638 (8.9566, -46.7237) -> (8.9871, -46.7096)
  line L1639 (8.9871, -46.7096) -> (9.0196, -46.6959)
  line L1640 (9.0196, -46.6959) -> (9.0542, -46.6827)
  line L1641 (8.8777, -46.7683) -> (8.9019, -46.7531)
  line L1642 (9.0542, -44.4235) -> (11, -45.1317)
  line L1643 (9.0542, -46.6827) -> (11, -45.9745)
  line L1644 (11, -45.1317) -> (11, -45.5531)
  line L1645 (11, -45.9745) -> (11, -45.5531)
  line L1646 (8.8777, -43.6267) -> (8.9019, -43.6115)
  line L1647 (9.0542, -41.2819) -> (11, -41.9901)
  line L1648 (9.0196, -43.5543) -> (9.0542, -43.5411)
  line L1649 (9.0542, -43.5411) -> (11, -42.8329)
  line L1650 (11, -42.8329) -> (11, -42.4115)
  line L1651 (11, -41.9901) -> (11, -42.4115)
  line L1652 (8.7511, -44.1729) -> (8.7542, -44.19)
  line L1653 (8.7511, -43.7917) -> (8.7542, -43.7746)
  line L1654 (8.7542, -43.7746) -> (8.7595, -43.7575)
  line L1655 (8.7595, -43.7575) -> (8.7669, -43.7406)
  line L1656 (8.7669, -43.7406) -> (8.7764, -43.7237)
  line L1657 (8.9871, -41.255) -> (9.0196, -41.2687)
  line L1658 (8.9871, -43.568) -> (9.0196, -43.5543)
  line L1659 (8.9566, -43.5821) -> (8.9871, -43.568)
  line L1660 (8.9282, -43.5966) -> (8.9566, -43.5821)
  line L1661 (8.8556, -43.6423) -> (8.8777, -43.6267)
  line L1662 (8.8355, -43.6581) -> (8.8556, -43.6423)
  line L1663 (8.8176, -43.6742) -> (8.8355, -43.6581)
  line L1664 (8.8018, -43.6905) -> (8.8176, -43.6742)
  line L1665 (8.788, -43.707) -> (8.8018, -43.6905)
  line L1666 (8.7764, -43.7237) -> (8.788, -43.707)
  line L1667 (8.7542, -44.19) -> (8.7595, -44.2071)
  line L1668 (8.9019, -43.6115) -> (8.9282, -43.5966)
  line L1669 (8.8018, -41.1325) -> (8.8176, -41.1488)
  line L1670 (8.8176, -41.1488) -> (8.8355, -41.1649)
  line L1671 (8.8355, -41.1649) -> (8.8556, -41.1807)
  line L1672 (8.8556, -41.1807) -> (8.8777, -41.1963)
  line L1673 (8.8777, -41.1963) -> (8.9019, -41.2115)
  line L1674 (8.9019, -41.2115) -> (8.9282, -41.2264)
  line L1675 (8.9282, -41.2264) -> (8.9566, -41.2409)
  line L1676 (9.0196, -41.2687) -> (9.0542, -41.2819)
  line L1677 (8.9566, -41.2409) -> (8.9871, -41.255)
  line L1678 (8.7764, -40.5821) -> (8.788, -40.5654)
  line L1679 (8.7669, -40.599) -> (8.7764, -40.5821)
  line L1680 (8.7595, -40.6159) -> (8.7669, -40.599)
  line L1681 (8.788, -40.5654) -> (8.8018, -40.5489)
  line L1682 (8.9282, -40.455) -> (8.9566, -40.4405)
  line L1683 (8.9019, -40.4699) -> (8.9282, -40.455)
  line L1684 (8.8777, -40.4851) -> (8.9019, -40.4699)
  line L1685 (8.8355, -40.5165) -> (8.8556, -40.5007)
  line L1686 (8.8176, -40.5326) -> (8.8355, -40.5165)
  line L1687 (8.8018, -40.5489) -> (8.8176, -40.5326)
  line L1688 (8.7595, -41.0655) -> (8.7669, -41.0824)
  line L1689 (8.7669, -41.0824) -> (8.7764, -41.0993)
  line L1690 (8.7764, -41.0993) -> (8.788, -41.116)
  line L1691 (8.788, -41.116) -> (8.8018, -41.1325)
  line L1692 (8.8556, -40.5007) -> (8.8777, -40.4851)
  line L1693 (9.0542, -38.1403) -> (11, -38.8485)
  line L1694 (8.9566, -40.4405) -> (8.9871, -40.4264)
  line L1695 (8.9871, -40.4264) -> (9.0196, -40.4128)
  line L1696 (9.0196, -40.4128) -> (9.0542, -40.3995)
  line L1697 (9.0542, -40.3995) -> (11, -39.6913)
  line L1698 (11, -39.6913) -> (11, -39.2699)
  line L1699 (11, -38.8485) -> (11, -39.2699)
  line L1700 (8.9871, -38.1134) -> (9.0196, -38.1271)
  line L1701 (9.0196, -38.1271) -> (9.0542, -38.1403)
  line L1702 (8.9566, -38.0993) -> (8.9871, -38.1134)
  line L1703 (8.9282, -38.0848) -> (8.9566, -38.0993)
  line L1704 (8.9019, -38.0699) -> (8.9282, -38.0848)
  line L1705 (8.8777, -38.0547) -> (8.9019, -38.0699)
  line L1706 (8.8556, -38.0392) -> (8.8777, -38.0547)
  line L1707 (8.8355, -38.0233) -> (8.8556, -38.0392)
  line L1708 (8.8176, -38.0072) -> (8.8355, -38.0233)
  line L1709 (8.8018, -37.9909) -> (8.8176, -38.0072)
  line L1710 (8.788, -37.9744) -> (8.8018, -37.9909)
  line L1711 (8.7764, -37.9577) -> (8.788, -37.9744)
  line L1712 (8.7542, -37.9068) -> (8.7595, -37.9239)
  line L1713 (8.7511, -37.8897) -> (8.7542, -37.9068)
  line L1714 (8.75, -37.8726) -> (8.7511, -37.8897)
  line L1715 (8.75, -37.6991) -> (8.75, -37.8726)
  line L1716 (8.75, -28.4478) -> (8.7511, -28.465)
  line L1717 (8.75, -28.2743) -> (8.75, -28.4478)
  line L1718 (8.75, -28.1008) -> (8.7511, -28.0837)
  line L1719 (8.75, -25.3062) -> (8.7511, -25.3234)
  line L1720 (8.75, -25.1327) -> (8.75, -25.3062)
  line L1721 (8.75, -28.2743) -> (8.75, -28.1008)
  line L1722 (8.8018, -47.4157) -> (8.8176, -47.432)
  line L1723 (8.8176, -47.432) -> (8.8355, -47.4481)
  line L1724 (8.8556, -47.4639) -> (8.8777, -47.4795)
  line L1725 (8.8777, -47.4795) -> (8.9019, -47.4947)
  line L1726 (8.9019, -47.4947) -> (8.9282, -47.5096)
  line L1727 (8.9282, -47.5096) -> (8.9566, -47.5241)
  line L1728 (8.9566, -47.5241) -> (8.9871, -47.5382)
  line L1729 (8.9871, -47.5382) -> (9.0196, -47.5518)
  line L1730 (9.0196, -47.5518) -> (9.0542, -47.5651)
  line L1731 (8.8355, -47.4481) -> (8.8556, -47.4639)
  line L1732 (8.7669, -21.7494) -> (8.7764, -21.7326)
  line L1733 (8.75, -25.1327) -> (7.9383, -25.1327)
  line L1734 (8.7595, -21.7664) -> (8.7669, -21.7494)
  line L1735 (8.75, -18.8496) -> (8.75, -18.6761)
  line L1736 (8.75, -18.6761) -> (8.7511, -18.6589)
  line L1737 (8.7511, -18.6589) -> (8.7542, -18.6418)
  line L1738 (8.7542, -18.6418) -> (8.7595, -18.6248)
  line L1739 (8.7595, -18.6248) -> (8.7669, -18.6078)
  line L1740 (8.7669, -18.6078) -> (8.7764, -18.591)
  line L1741 (8.7764, -18.591) -> (8.788, -18.5743)
  line L1742 (8.788, -18.5743) -> (8.8018, -18.5578)
  line L1743 (8.8018, -18.5578) -> (8.8176, -18.5414)
  line L1744 (8.8176, -18.5414) -> (8.8355, -18.5253)
  line L1745 (8.8355, -18.5253) -> (8.8556, -18.5095)
  line L1746 (8.8556, -18.5095) -> (8.8777, -18.494)
  line L1747 (8.8777, -18.494) -> (8.9019, -18.4787)
  line L1748 (8.9019, -18.4787) -> (8.9282, -18.4639)
  line L1749 (9.0542, -16.1491) -> (11, -16.8573)
  line L1750 (8.9282, -18.4639) -> (8.9566, -18.4494)
  line L1751 (8.9566, -18.4494) -> (8.9871, -18.4353)
  line L1752 (8.9871, -18.4353) -> (9.0196, -18.4216)
  line L1753 (9.0196, -18.4216) -> (9.0542, -18.4084)
  line L1754 (11, -16.8573) -> (11, -17.2788)
  line L1755 (11, -17.7002) -> (11, -17.2788)
  line L1756 (9.0542, -18.4084) -> (11, -17.7002)
  line L1757 (8.8556, -16.048) -> (8.8777, -16.0635)
  line L1758 (8.8777, -16.0635) -> (8.9019, -16.0788)
  line L1759 (8.9019, -16.0788) -> (8.9282, -16.0936)
  line L1760 (8.9282, -16.0936) -> (8.9566, -16.1082)
  line L1761 (8.9566, -16.1082) -> (8.9871, -16.1222)
  line L1762 (9.0196, -16.1359) -> (9.0542, -16.1491)
  line L1763 (8.9871, -16.1222) -> (9.0196, -16.1359)
  line L1764 (8.8355, -16.0322) -> (8.8556, -16.048)
  line L1765 (8.8018, -15.9998) -> (8.8176, -16.0161)
  line L1766 (8.788, -15.9832) -> (8.8018, -15.9998)
  line L1767 (8.7764, -15.9665) -> (8.788, -15.9832)
  line L1768 (8.7669, -15.9497) -> (8.7764, -15.9665)
  line L1769 (8.7595, -15.9327) -> (8.7669, -15.9497)
  line L1770 (8.8176, -16.0161) -> (8.8355, -16.0322)
  line L1771 (8.8176, -15.3998) -> (8.8355, -15.3838)
  line L1772 (8.8018, -15.4162) -> (8.8176, -15.3998)
  line L1773 (8.788, -15.4327) -> (8.8018, -15.4162)
  line L1774 (8.7764, -15.4494) -> (8.788, -15.4327)
  line L1775 (8.7669, -15.4662) -> (8.7764, -15.4494)
  line L1776 (8.75, -15.8814) -> (8.7511, -15.8986)
  line L1777 (8.7511, -15.8986) -> (8.7542, -15.9157)
  line L1778 (8.7542, -15.9157) -> (8.7595, -15.9327)
  line L1779 (8.7595, -15.4832) -> (8.7669, -15.4662)
  line L1780 (8.9566, -12.9666) -> (8.9871, -12.9807)
  line L1781 (8.9871, -12.9807) -> (9.0196, -12.9943)
  line L1782 (9.0196, -12.9943) -> (9.0542, -13.0075)
  line L1783 (9.0542, -15.2668) -> (11, -14.5586)
  line L1784 (9.0542, -13.0075) -> (11, -13.7157)
  line L1785 (11, -14.5586) -> (11, -14.1372)
  line L1786 (11, -13.7157) -> (11, -14.1372)
  line L1787 (8.8355, -15.3838) -> (8.8556, -15.3679)
  line L1788 (8.8556, -15.3679) -> (8.8777, -15.3524)
  line L1789 (8.8777, -15.3524) -> (8.9019, -15.3372)
  line L1790 (8.9019, -15.3372) -> (8.9282, -15.3223)
  line L1791 (8.9282, -15.3223) -> (8.9566, -15.3078)
  line L1792 (8.9566, -15.3078) -> (8.9871, -15.2937)
  line L1793 (8.9871, -15.2937) -> (9.0196, -15.28)
  line L1794 (9.0196, -15.28) -> (9.0542, -15.2668)
  line L1795 (8.9282, -12.9521) -> (8.9566, -12.9666)
  line L1796 (8.9019, -12.9372) -> (8.9282, -12.9521)
  line L1797 (8.8777, -12.922) -> (8.9019, -12.9372)
  line L1798 (8.8355, -12.8906) -> (8.8556, -12.9064)
  line L1799 (8.8176, -12.8745) -> (8.8355, -12.8906)
  line L1800 (8.8018, -12.8582) -> (8.8176, -12.8745)
  line L1801 (8.788, -12.8416) -> (8.8018, -12.8582)
  line L1802 (8.8556, -12.9064) -> (8.8777, -12.922)
  line L1803 (8.7764, -12.8249) -> (8.788, -12.8416)
  line L1804 (8.7669, -12.8081) -> (8.7764, -12.8249)
  line L1805 (8.7595, -12.7911) -> (8.7669, -12.8081)
  line L1806 (8.7542, -12.7741) -> (8.7595, -12.7911)
  line L1807 (8.75, -12.7399) -> (8.7511, -12.757)
  line L1808 (8.75, -12.5664) -> (8.75, -12.7399)
  line L1809 (8.7511, -12.757) -> (8.7542, -12.7741)
  line L1810 (8.75, -21.9911) -> (8.75, -21.8177)
  line L1811 (8.75, -21.8177) -> (8.7511, -21.8005)
  line L1812 (8.7511, -21.8005) -> (8.7542, -21.7834)
  line L1813 (8.75, -15.708) -> (8.75, -15.8814)
  line L1814 (8.75, -15.708) -> (8.75, -15.5345)
  line L1815 (8.75, -15.5345) -> (8.7511, -15.5173)
  line L1816 (8.7511, -15.5173) -> (8.7542, -15.5002)
  line L1817 (8.7542, -15.5002) -> (8.7595, -15.4832)
  line L1818 (8.7669, -37.9408) -> (8.7764, -37.9577)
  line L1819 (8.7595, -37.9239) -> (8.7669, -37.9408)
  line L1820 (8.75, -37.5256) -> (8.7511, -37.5085)
  line L1821 (8.7511, -37.5085) -> (8.7542, -37.4914)
  line L1822 (8.7542, -37.4914) -> (8.7595, -37.4743)
  line L1823 (8.7595, -37.4743) -> (8.7669, -37.4574)
  line L1824 (8.7669, -37.4574) -> (8.7764, -37.4405)
  line L1825 (8.7764, -37.4405) -> (8.788, -37.4238)
  line L1826 (8.8018, -37.4073) -> (8.8176, -37.391)
  line L1827 (8.8176, -37.391) -> (8.8355, -37.3749)
  line L1828 (8.8355, -37.3749) -> (8.8556, -37.3591)
  line L1829 (8.788, -37.4238) -> (8.8018, -37.4073)
  line L1830 (8.75, -37.6991) -> (8.75, -37.5256)
  line L1831 (8.8556, -31.756) -> (8.8777, -31.7715)
  line L1832 (8.8355, -31.7401) -> (8.8556, -31.756)
  line L1833 (8.8176, -31.724) -> (8.8355, -31.7401)
  line L1834 (8.8018, -31.7077) -> (8.8176, -31.724)
  line L1835 (8.788, -31.6912) -> (8.8018, -31.7077)
  line L1836 (8.7764, -31.6745) -> (8.788, -31.6912)
  line L1837 (8.7669, -31.6577) -> (8.7764, -31.6745)
  line L1838 (8.7669, -31.1742) -> (8.7764, -31.1574)
  line L1839 (8.7595, -31.1912) -> (8.7669, -31.1742)
  line L1840 (8.7542, -31.2082) -> (8.7595, -31.1912)
  line L1841 (8.7511, -31.2253) -> (8.7542, -31.2082)
  line L1842 (8.75, -31.4159) -> (8.75, -31.2424)
  line L1843 (8.75, -31.4159) -> (8.75, -31.5894)
  line L1844 (8.75, -31.5894) -> (8.7511, -31.6065)
  line L1845 (8.7511, -31.6065) -> (8.7542, -31.6236)
  line L1846 (8.7542, -31.6236) -> (8.7595, -31.6407)
  line L1847 (8.75, -31.2424) -> (8.7511, -31.2253)
  line L1848 (8.8777, -31.0603) -> (8.9019, -31.0451)
  line L1849 (8.8176, -31.1078) -> (8.8355, -31.0917)
  line L1850 (8.8355, -31.0917) -> (8.8556, -31.0759)
  line L1851 (8.8556, -31.0759) -> (8.8777, -31.0603)
  line L1852 (8.8018, -31.1241) -> (8.8176, -31.1078)
  line L1853 (8.788, -31.1407) -> (8.8018, -31.1241)
  line L1854 (8.7764, -31.1574) -> (8.788, -31.1407)
  line L1855 (8.7595, -31.6407) -> (8.7669, -31.6577)
  line L1856 (8.9019, -31.0451) -> (8.9282, -31.0302)
  line L1857 (8.7511, -28.465) -> (8.7542, -28.4821)
  line L1858 (8.7542, -28.4821) -> (8.7595, -28.4991)
  line L1859 (8.7595, -28.4991) -> (8.7669, -28.5161)
  line L1860 (8.7669, -28.5161) -> (8.7764, -28.5329)
  line L1861 (8.7764, -28.5329) -> (8.788, -28.5496)
  line L1862 (8.788, -28.5496) -> (8.8018, -28.5661)
  line L1863 (8.8018, -28.5661) -> (8.8176, -28.5825)
  line L1864 (8.8176, -28.5825) -> (8.8355, -28.5985)
  line L1865 (8.8355, -28.5985) -> (8.8556, -28.6144)
  line L1866 (8.8556, -28.6144) -> (8.8777, -28.6299)
  line L1867 (8.8777, -28.6299) -> (8.9019, -28.6451)
  line L1868 (8.9019, -28.6451) -> (8.9282, -28.66)
  line L1869 (8.7764, -28.0158) -> (8.788, -27.9991)
  line L1870 (8.788, -27.9991) -> (8.8018, -27.9825)
  line L1871 (8.7669, -28.0326) -> (8.7764, -28.0158)
  line L1872 (8.7595, -28.0496) -> (8.7669, -28.0326)
  line L1873 (8.7542, -28.0666) -> (8.7595, -28.0496)
  line L1874 (8.7511, -28.0837) -> (8.7542, -28.0666)
  line L1875 (9.0196, -27.8464) -> (9.0542, -27.8332)
  line L1876 (8.9871, -27.86) -> (9.0196, -27.8464)
  line L1877 (8.9566, -27.8741) -> (8.9871, -27.86)
  line L1878 (8.9282, -27.8886) -> (8.9566, -27.8741)
  line L1879 (8.9019, -27.9035) -> (8.9282, -27.8886)
  line L1880 (8.8777, -27.9188) -> (8.9019, -27.9035)
  line L1881 (8.8556, -27.9343) -> (8.8777, -27.9188)
  line L1882 (8.8355, -27.9501) -> (8.8556, -27.9343)
  line L1883 (8.8176, -27.9662) -> (8.8355, -27.9501)
  line L1884 (8.8018, -27.9825) -> (8.8176, -27.9662)
  line L1885 (9.0542, -27.8332) -> (11, -27.125)
  line L1886 (8.7669, -25.3745) -> (8.7764, -25.3913)
  line L1887 (8.7595, -25.3575) -> (8.7669, -25.3745)
  line L1888 (8.7542, -25.3405) -> (8.7595, -25.3575)
  line L1889 (8.7511, -25.3234) -> (8.7542, -25.3405)
  line L1890 (9.0542, -25.5739) -> (11, -26.2821)
  line L1891 (11, -26.2821) -> (11, -26.7035)
  line L1892 (11, -27.125) -> (11, -26.7035)
  line L1893 (9.0196, -25.5607) -> (9.0542, -25.5739)
  line L1894 (8.9871, -25.547) -> (9.0196, -25.5607)
  line L1895 (8.9566, -25.5329) -> (8.9871, -25.547)
  line L1896 (8.9282, -25.5184) -> (8.9566, -25.5329)
  line L1897 (8.9019, -25.5035) -> (8.9282, -25.5184)
  line L1898 (8.8777, -25.4883) -> (8.9019, -25.5035)
  line L1899 (8.8556, -25.4728) -> (8.8777, -25.4883)
  line L1900 (8.8355, -25.457) -> (8.8556, -25.4728)
  line L1901 (8.8176, -25.4409) -> (8.8355, -25.457)
  line L1902 (8.8018, -25.4245) -> (8.8176, -25.4409)
  line L1903 (8.788, -25.408) -> (8.8018, -25.4245)
  line L1904 (8.7764, -25.3913) -> (8.788, -25.408)
  line L1905 (9.0196, -0.428) -> (9.0542, -0.4412)
  line L1906 (8.9871, -0.4143) -> (9.0196, -0.428)
  line L1907 (8.9566, -0.4002) -> (8.9871, -0.4143)
  line L1908 (8.9282, -0.3857) -> (8.9566, -0.4002)
  line L1909 (8.9019, -0.3708) -> (8.9282, -0.3857)
  line L1910 (8.8777, -0.3556) -> (8.9019, -0.3708)
  line L1911 (8.8556, -0.34) -> (8.8777, -0.3556)
  line L1912 (8.8355, -0.3242) -> (8.8556, -0.34)
  line L1913 (8.8176, -0.3081) -> (8.8355, -0.3242)
  line L1914 (8.8018, -0.2918) -> (8.8176, -0.3081)
  line L1915 (8.75, -3.1416) -> (8.75, -2.9681)
  line L1916 (8.75, -3.1416) -> (8.75, -3.3151)
  line L1917 (8.75, -3.3151) -> (8.7511, -3.3322)
  line L1918 (8.7511, -3.3322) -> (8.7542, -3.3493)
  line L1919 (8.7542, -3.3493) -> (8.7595, -3.3664)
  line L1920 (8.788, -2.8663) -> (8.8018, -2.8498)
  line L1921 (8.8018, -2.8498) -> (8.8176, -2.8335)
  line L1922 (8.75, -2.9681) -> (8.7511, -2.951)
  line L1923 (8.7511, -2.951) -> (8.7542, -2.9339)
  line L1924 (8.7542, -2.9339) -> (8.7595, -2.9168)
  line L1925 (8.7595, -2.9168) -> (8.7669, -2.8999)
  line L1926 (8.7764, -2.883) -> (8.788, -2.8663)
  line L1927 (8.8176, -2.8335) -> (8.8355, -2.8174)
  line L1928 (8.8355, -2.8174) -> (8.8556, -2.8016)
  line L1929 (8.8556, -2.8016) -> (8.8777, -2.786)
  line L1930 (8.8777, -2.786) -> (8.9019, -2.7708)
  line L1931 (8.9019, -2.7708) -> (8.9282, -2.7559)
  line L1932 (8.9282, -2.7559) -> (8.9566, -2.7414)
  line L1933 (8.7669, -2.8999) -> (8.7764, -2.883)
  line L1934 (8.75, -3.1416) -> (7.1265, -3.1416)
  line L1935 (8.8777, -5.9276) -> (8.9019, -5.9124)
  line L1936 (8.9019, -5.9124) -> (8.9282, -5.8975)
  line L1937 (8.9282, -5.8975) -> (8.9566, -5.883)
  line L1938 (8.75, -6.2832) -> (8.75, -6.1097)
  line L1939 (8.75, -6.1097) -> (8.7511, -6.0926)
  line L1940 (8.7511, -6.0926) -> (8.7542, -6.0755)
  line L1941 (8.7542, -6.0755) -> (8.7595, -6.0584)
  line L1942 (8.7595, -6.0584) -> (8.7669, -6.0415)
  line L1943 (8.7669, -6.0415) -> (8.7764, -6.0246)
  line L1944 (8.7764, -6.0246) -> (8.788, -6.0079)
  line L1945 (8.788, -6.0079) -> (8.8018, -5.9914)
  line L1946 (8.8018, -5.9914) -> (8.8176, -5.9751)
  line L1947 (8.8176, -5.9751) -> (8.8355, -5.959)
  line L1948 (8.8355, -5.959) -> (8.8556, -5.9431)
  line L1949 (8.8556, -5.9431) -> (8.8777, -5.9276)
  line L1950 (8.9566, -5.883) -> (8.9871, -5.8689)
  line L1951 (8.9871, -5.8689) -> (9.0196, -5.8552)
  line L1952 (9.0196, -5.8552) -> (9.0542, -5.842)
  line L1953 (9.0542, -5.842) -> (11, -5.1338)
  line L1954 (11, -5.1338) -> (11, -4.7124)
  line L1955 (9.0542, -3.5828) -> (11, -4.291)
  line L1956 (8.9871, -3.5559) -> (9.0196, -3.5695)